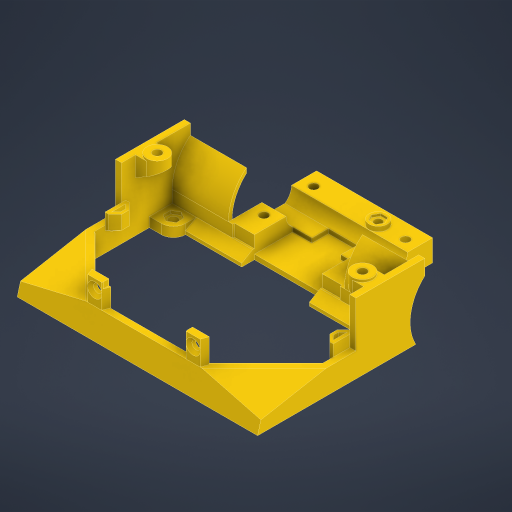
# Autodesk Inventor part: body
Saved by Autodesk Inventor 2024 (Build 280153000, 153)
## iProperties
Created: 2024-01-31
Part Number: body
Material: Všeobecné
Document SubType Name: Modeling
Designer: Simak
Density: 1 g/cm^3
Appearance: Výchozí
Author: Simak
Autodesk Inventor part; units mm, degrees
ref_plane "YZ Plane" through (0, 0, 0) normal (1, 0, 0) x (0, 1, 0)
ref_plane "XZ Plane" through (0, 0, 0) normal (0, 1, 0) x (-1, 0, 0)
ref_plane "XY Plane" through (0, 0, 0) normal (0, 0, 1) x (1, 0, 0)
sketch "Náčrt2" plane through (0, 0, 0) normal (0, 1, 0) x (-1, 0, 0)
  line L0 (0, 49.75) -> (-49.75, 49.75)
  line L1 (-49.75, 49.75) -> (-49.75, -49.75)
  line L2 (-49.75, -49.75) -> (0, -49.75)
  line L3 (-49.75, 49.75) -> (0, 0) construction
  line L4 (0, 0) -> (-49.75, -49.75) construction
  line L5 (-47.25, 49.75) -> (-47.25, -17.75)
  line L6 (-47.25, -17.75) -> (-49.75, -17.75)
  line L7 (0, 49.75) -> (0, -49.75)
  dimension "d0" = 99.5
  dimension "d1" = 67.5
  dimension "d2" = 2.5
  constraints: 16 end point, 5 perpendicular, 2 point on line, 2 vertical, 2 vertical alignment, 1 horizontal
  measures "d0" distance of L0.end L1.end
  measures "d1" distance of L5.start L5.end
  measures "d2" distance of L5.end L6.end
extrude "Vysunutí1" add sketch "Náčrt2" along normal blind 10 contours L5 L6 L1 L0
sketch "Náčrt3" plane through (49.75, 0, 49.75) normal (1, 0, 0) x (0, 0, -1)
  line L0 (67.5, 0) -> (0, 0) projected
  line L1 (67.5, 10) -> (0, 10) projected
  line L2 (0, 0) -> (0, 10) projected
  line L3 (0, 0) -> (0, -5)
  line L4 (0, -5) -> (67.5, -5) construction
  line L5 (67.5, -5) -> (67.5, 0) construction
  line L6 (0, -5) -> (4.0192, 10)
  point P0 (49.75, 0)
  point P1 (1.3397, 0)
  dimension "d8" = 5
  dimension "d9" = 75
  constraints: 8 end point, 2 perpendicular, 1 point on line, 1 vertical
  measures "d8" distance of L4.end L0.start
  measures "d9" angle of L4 L6
extrude "Vysunutí2" cut sketch "Náčrt3" against normal blind 10 contours L0 L2 L1 L6
sketch "Náčrt4" plane through (49.75, 0, -17.75) normal (1, 0, 0) x (0, 0, -1)
  line L0 (0, 10) -> (-63.4808, 10) projected
  line L1 (-60.8926, 10) -> (-63.5721, 0)
  line L2 (0, 0) -> (-66.1603, 0) projected
  line L3 (-63.4808, 10) -> (-66.1603, 0) projected
  point P0 (-17.75, 0)
  dimension "d10" = 2.5
  constraints: 2 end point, 2 point on line, 1 parallel
  measures "d10" distance between parallel lines of L3 L1
extrude "Vysunutí3" add sketch "Náčrt4" against normal up to surface (49.75 mm away)
sketch "Náčrt5" plane through (49.75, 0, -17.75) normal (1, 0, 0) x (0, 0, -1)
  line L0 (-63.4808, 10) -> (0, 10) projected
  line L1 (-25.4808, 10) -> (0, 10)
  line L2 (0, 10) -> (0, 29)
  line L3 (0, 29) -> (-25.4808, 29)
  line L4 (-25.4808, 29) -> (-25.4808, 10)
  point P0 (-17.75, 0)
  dimension "d13" = 38
  dimension "d14" = 19
  constraints: 8 end point, 2 parallel, 1 horizontal, 1 perpendicular, 1 point on line
  measures "d13" distance from line of L4 L0.start
  measures "d14" distance of L3.end L1.start
extrude "Vysunutí4" add sketch "Náčrt5" against normal up to surface (2.5 mm away)
sketch "Náčrt6" plane through (47.25, 0, -17.75) normal (-1, 0, 0) x (0, 0, 1)
  line L0 (63.5721, 0) -> (60.8926, 10) projected
  line L1 (55.5721, 1) -> (63.5721, 1)
  line L2 (63.5721, 1) -> (63.5721, 0)
  line L3 (63.5721, 0) -> (55.5721, 0)
  line L4 (55.5721, 0) -> (55.5721, 1)
  point P0 (17.75, 0)
  dimension "d17" = 1
  dimension "d18" = 8
  constraints: 8 end point, 2 parallel, 1 horizontal, 1 perpendicular
  measures "d17" distance of L3.end L1.start
  measures "d18" distance of L1.start L1.end
extrude "Vysunutí5" add sketch "Náčrt6" along normal up to surface (47.25 mm away)
sketch "Náčrt7" plane through (47.25, 0, -17.75) normal (-1, 0, 0) x (0, 0, 1)
  line L0 (60.8926, 10) -> (63.3041, 1) projected
  line L1 (62.7682, 3) -> (63.3041, 3)
  line L2 (63.3041, 3) -> (63.3041, 1)
  line L3 (63.3041, 1) -> (62.7682, 1)
  line L4 (62.7682, 1) -> (62.7682, 3)
  point P0 (17.75, 0)
  dimension "d21" = 2
  constraints: 8 end point, 2 parallel, 1 horizontal, 1 perpendicular, 1 point on line
  measures "d21" distance of L3.end L1.start
extrude "Vysunutí6" cut sketch "Náčrt7" along normal up to surface (47.25 mm away) contours L1 L2 L0
sketch "Náčrt8" plane through (0, 10, 0) normal (0, 1, 0) x (1, 0, 0)
  line L0 (49.75, -45.7308) -> (49.75, -7.7308) projected
  point P0 (0, 0)
  point P1 (24.0355, -45.7308)
  point P2 (49.75, -20.0163)
  dimension "d24" = 25.7145
  dimension "d25" = 25.7145
  constraints: 1 horizontal alignment, 1 point on line, 1 vertical alignment
  measures "d24" distance from line of L0 point (24.036, -45.731)
  measures "d25" distance of L0.start point (49.75, -20.016)
sketch "Náčrt9" plane through (49.75, 0, 48.4103) normal (1, 0, 0) x (0, 0, -1)
  line L0 (1.3397, 5) -> (0, 0) construction
  line L1 (2.6795, 10) -> (5.2677, 10) projected
  line L2 (1.3397, 5) -> (2.6795, 10) construction
  point P0 (48.4103, 0)
  constraints: 4 end point, 2 collinear
ref_plane "Pracovní rovina1" through (24.0355, 10, 45.7308) normal (-0.1788076, -0.9674997, -0.1788076) x (0.7071068, 0, -0.7071068)
sketch "Náčrt10" plane through (24.0355, 10, 45.7308) normal (-0.1788076, -0.9674997, -0.1788076) x (0.7071068, 0, -0.7071068)
  line L0 (18.1829, 17.5919) -> (-16.9957, -16.4433) projected
  line L1 (0, 0) -> (17.2355, 19.7728)
  line L2 (18.1829, 17.5919) -> (16.2882, 21.9538) projected
  line L3 (17.2355, 19.7728) -> (36.3657, 0)
  line L4 (0, 0) -> (36.3657, 0)
  point P0 (15.3408, -45.2002)
  point P1 (17.2355, 19.7728)
  point P2 (36.3657, 0)
  constraints: 6 end point, 1 coincident, 1 horizontal, 1 midpoint
extrude "Vysunutí7" cut sketch "Náčrt10" against normal blind 10
sketch "Náčrt11" plane through (24.0355, 10, 45.7308) normal (0.1788076, 0.9674997, 0.1788076) x (0.6841256, -0.2528721, 0.6841256)
  line L0 (0, 3.6603) -> (15.8603, 17.4853) projected
  line L1 (0, 0) -> (0, 3.6603) projected
  line L2 (19.7728, 17.2355) -> (0, 0) projected
  line L3 (0, 36.3657) -> (19.7728, 17.2355) projected
  line L4 (0, 32.8302) -> (0, 36.3657) projected
  line L5 (15.8603, 17.4853) -> (0, 32.8302) projected
  line L6 (0, 3.6603) -> (0, 32.8302)
  point P0 (-45.2002, 15.3408)
  constraints: 2 end point, 1 vertical
extrude "Vysunutí8" add sketch "Náčrt11" against normal blind 1.5
sketch "Náčrt13" plane through (23.7673, 8.5488, 45.4626) normal (-0.1788076, -0.9674997, -0.1788076) x (0.7071068, 0, -0.7071068)
  line L0 (17.1763, 16.5718) -> (33.2095, 0) projected
  line L1 (2.731, 0) -> (17.1763, 16.5718) projected
  line L2 (2.731, 0) -> (33.2095, 0) projected
  line L3 (33.2095, 0) -> (35.5528, -2.422)
  line L4 (43.2852, -10.1152) -> (32.8302, 0) projected
  line L5 (35.5528, -2.422) -> (0.6198, -2.422)
  line L6 (0.6198, -2.422) -> (2.731, 0)
  point P0 (15.3408, -45.2002)
  point P1 (39.216, -6.1783)
  point P2 (2.731, 0)
  point P3 (35.3336, -2.422)
  dimension "d30" = 2.422
  constraints: 6 end point, 2 collinear, 2 point on line, 1 horizontal
  measures "d30" distance between parallel lines of L2 L5
extrude "Vysunutí9" add sketch "Náčrt13" against normal up to surface contours L3 L5 L4 L2 | L2 L4 L5 L6 surface through (48.5, 10, 16) normal (0, 1, 0)
sketch "Náčrt14" plane through (0, 0, 0) normal (0, -1, 0) x (1, 0, 0)
  line L0 (47.25, 37.8221) -> (0, 37.8221) projected
  line L1 (44.25, 37.8221) -> (36.75, 37.8221)
  line L2 (36.75, 37.8221) -> (36.75, 41.8041)
  line L3 (44.25, 41.8041) -> (44.25, 37.8221)
  line L4 (49.75, 48.4103) -> (49.75, -17.75) projected
  line L5 (49.75, 48.4103) -> (0, 48.4103) projected
  arc A0 (44.25, 41.8041) -> (36.75, 41.8041) centre (40.5, 41.8041) ccw
  line L6 (47.25, 45.5541) -> (0, 45.5541) projected
  line L7 (47.25, 45.5541) -> (0, 45.5541) projected
  point P0 (0, 0)
  point P1 (36.75, 37.8221)
  point P2 (40.5, 45.5541)
  dimension "d33" = 5.5
  dimension "d35" = 7.5
  constraints: 6 end point, 3 point on circle, 2 point on line, 2 tangent, 1 centre point, 1 horizontal, 1 parallel, 1 perpendicular
  measures "d33" distance between parallel lines of L4 L3
  measures "d35" distance of L2.end L3.start
extrude "Vysunutí10" cut sketch "Náčrt14" against normal up to surface (1 mm away)
sketch "Náčrt15" plane through (47.25, 0, -17.75) normal (-1, 0, 0) x (0, 0, 1)
  circle A0 centre (-15.5, 9) radius 18.5
  line L0 (0, 0) -> (0, 29) projected
  line L1 (0, 0) -> (55.5721, 0) projected
  circle A1 centre (-15.5, 9) radius 20
  line L2 (-3, 24.6125) -> (-3, 22.6382)
  point P0 (17.75, 0)
  point P1 (0, 21.6392)
  point P2 (0, 19.0995)
  point P3 (0.6632, 0)
  point P4 (2.3606, 0)
  point P5 (0, 0.876)
  dimension "d39" = 37
  dimension "d41" = 1.5
  dimension "d38" = 15.5
  dimension "d44" = 9
  dimension "d47" = 6
  constraints: 2 end point, 1 vertical, 6 other
  measures "d38" distance from line of L0 point (-15.5, 9)
  measures "d44" distance from line of L1 point (-15.5, 9)
extrude "Vysunutí11" cut sketch "Náčrt15" against normal up to surface (2.5 mm away) contours A0 L1 L0 | L0 L1 A0
extrude "Vysunutí12" add sketch "Náčrt15" along normal blind 25 contours A0 L0 A1 L1 | A0 L2 A1 L0
sketch "Náčrt16" plane through (49.75, 29, 7.7308) normal (0, 1, 0) x (1, 0, 0)
  line L0 (-2.5, 28.4808) -> (-2.5, 25.4808) projected
  line L1 (0, 25.4808) -> (-2.5, 25.4808) projected
  line L2 (-2.5, 25.4808) -> (0, 25.4808)
  line L3 (0, 25.4808) -> (0, 28.4808)
  line L4 (0, 28.4808) -> (-2.5, 28.4808)
  line L5 (-2.5, 28.4808) -> (-2.5, 25.4808)
  point P0 (-49.75, 7.7308)
  point P1 (-2.5, 23.1202)
  constraints: 8 end point, 4 parallel, 1 horizontal, 1 perpendicular
extrude "Vysunutí13" add sketch "Náčrt16" against normal up to surface round surface about axis through (47.25, 9, -33.25) along (1, 0, 0) radius 18.5 far side no
sketch "Náčrt18" plane through (47.25, 29, 7.7308) normal (0, 1, 0) x (1, 0, 0)
  circle A0 centre (-4.75, 10) radius 4.25
  line L0 (0, 28.4808) -> (0, 0) projected
  line L1 (2.5, 0) -> (0, 0) projected
  line L2 (2.5, 28.4808) -> (2.5, 0) projected
  line L3 (2.5, 28.4808) -> (0, 28.4808) projected
  line L4 (-4.75, 5.75) -> (0, 5.75)
  line L5 (-4.75, 14.25) -> (0, 14.25)
  circle A1 centre (-4.75, 10) radius 1.75
  point P0 (-47.25, 7.7308)
  dimension "d51" = 3.5
  dimension "d52" = 2.5
  dimension "d53" = 4.75
  dimension "d54" = 10
  constraints: 4 end point, 2 centre point, 2 point on circle, 2 point on line, 1 coincident, 1 horizontal, 1 parallel, 1 perpendicular, 1 tangent
  measures "d51" diameter of A1
  measures "d52" radial gap between concentric circles of A0 A1
  measures "d53" distance from line of L0 A0.centre
  measures "d54" distance from line of L1 A0.centre
extrude "Vysunutí14" add sketch "Náčrt18" against normal blind 3.5 contours A0 | A0 L5 L0 L4
extrude "Vysunutí15" add sketch "Náčrt18" along normal blind 1 contours A0
sketch "Náčrt20" plane through (0, 0, 0) normal (0, -1, 0) x (1, 0, 0)
  line L0 (0, -14) -> (24, -14)
  line L1 (24, -14) -> (24, -49.75)
  line L2 (24, -49.75) -> (0, -49.75)
  line L3 (0, -49.75) -> (0, -14)
  line L4 (22.25, -20.75) -> (49.75, -20.75) projected
  point P0 (0, 0)
  dimension "d63" = 29
  dimension "d82" = 14
  constraints: 8 end point, 2 parallel, 1 horizontal, 1 perpendicular, 1 vertical alignment
  measures "d63" distance between parallel lines of L4 L2
  measures "d82" distance from line of point (0, 0) L0
extrude "Vysunutí16" add sketch "Náčrt20" against normal blind 9
sketch "Náčrt21" plane through (24, 0, -17.0868) normal (1, 0, 0) x (0, 0, -1)
  line L0 (12.7467, 3.9) -> (19.5797, 3.9)
  line L1 (-2.3368, 9) -> (32.6632, 9) projected
  arc A0 (19.5797, 3.9) -> (22.3018, 9) centre (16.1632, 9) ccw
  arc A1 (10.0246, 9) -> (12.7467, 3.9) centre (16.1632, 9) ccw
  line L2 (32.6632, 0) -> (32.6632, 9) projected
  point P0 (-17.0868, 0)
  point P1 (-1.6973, 9)
  dimension "d66" = 5.1
  dimension "d67" = 16.5
  dimension "d68" = 6.833
  constraints: 4 point on circle, 2 centre point, 2 end point, 2 line through centre, 2 point on line, 1 coincident, 1 concentric, 1 horizontal
  measures "d66" distance between parallel lines of L0 L1
  measures "d67" distance from line of L2 A0.centre
  measures "d68" distance of L0.start L0.end
extrude "Vysunutí17" cut sketch "Náčrt21" against normal up to next
sketch "Náčrt23" plane through (24, 0, -49.75) normal (0, 0, -1) x (-1, 0, 0)
  line L0 (0, 3.9) -> (24, 3.9) projected
  line L1 (0, 3.9) -> (24, 3.9) projected
  line L2 (18, 3.9) -> (18, 9)
  line L3 (24, 0) -> (0, 0) projected
  line L4 (24, 0) -> (24, 9) projected
  line L5 (0, 9) -> (24, 9) projected
  line L6 (0, 0) -> (0, 9) projected
  point P0 (24, 0)
  dimension "d73" = 18
  constraints: 2 end point, 2 point on line, 1 perpendicular
  measures "d73" distance between parallel lines of L6 L2
extrude "Vysunutí19" cut sketch "Náčrt23" against normal up to surface (35.75 mm away) contours L2 L5 L4 L0
sketch "Náčrt49" plane through (6, 3.9, -49.75) normal (-1, 0, 0) x (0, 0, 1)
  arc A0 (10.3614, 5.1) -> (13.0835, 0) centre (16.5, 5.1) ccw projected
  line L0 (0, 5.1) -> (10.3614, 5.1) projected
  line L1 (0, 0) -> (0, 5.1) projected
  line L2 (0, 0) -> (13.0835, 0) projected
  point P0 (49.75, -3.9)
extrude "Vysunutí48" add sketch "Náčrt49" along normal up to surface (6 mm away)
sketch "Náčrt24" plane through (0, 9, 0) normal (0, 1, 0) x (1, 0, 0)
  line L0 (22.25, 14) -> (22.25, 20.75) projected
  line L1 (47.25, 15.3894) -> (24, 15.3894) projected
  line L2 (47.25, 20.75) -> (47.25, 15.3894) projected
  line L3 (47.25, 20.75) -> (22.25, 20.75) projected
  line L4 (6, 27.1114) -> (6, 14) projected
  line L5 (24, 14.75) -> (22.25, 14.75) projected
  line L6 (24, 27.1114) -> (6, 27.1114) projected
  line L7 (24, 29.8335) -> (6, 29.8335) projected
  line L8 (24, 36.6665) -> (24, 29.8335) projected
  line L9 (24, 36.6665) -> (0, 36.6665) projected
  line L10 (0, 14) -> (0, 36.6665) projected
  line L11 (6, 29.8335) -> (6, 14) projected
  line L12 (47.25, 13.25) -> (22.25, 13.25) projected
  line L13 (22.25, 20.75) -> (22.25, 13.25) projected
  line L14 (24, 14.75) -> (24, 13.25)
  line L15 (6, 29.8335) -> (0, 29.8335)
  line L16 (6, 36.6665) -> (6, 29.8335)
  line L17 (6, 36.6665) -> (0, 36.6665)
  line L18 (22.25, 14) -> (24, 14) projected
  line L19 (24, 14) -> (24, 15.3894) projected
  line L20 (6, 14) -> (0, 14) projected
  line L21 (22.25, 14.75) -> (22.25, 14) projected
  line L22 (24, 14.75) -> (24, 27.1114) projected
  line L23 (0, 39.3886) -> (24, 39.3886) projected
  line L24 (24, 39.3886) -> (24, 49.75) projected
  line L25 (24, 49.75) -> (0, 49.75) projected
  line L26 (6, 14) -> (22.25, 14) projected
  line L27 (14, 29.8335) -> (14, 14)
  line L28 (0, 49.75) -> (0, 39.3886) projected
  point P0 (0, 0)
  point P1 (22.25, 15.3894)
  point P2 (22.25, 15.3894)
  point P3 (22.25, 13.25)
  point P4 (24, 20.75)
  dimension "d84" = 10
  constraints: 10 end point, 5 perpendicular, 5 point on line
  measures "d84" distance between parallel lines of L22 L27
extrude "Vysunutí20" cut sketch "Náčrt24" along normal up to next contours L18 L14 L12 L13 | L0 L5 L14 L18 | L0 L3 L22 L19 L5
extrude "Vysunutí21" cut sketch "Náčrt24" against normal blind 7 contours L26 L4 L6 L27 | L20 L10 L15 L11 L4 | L6 L11 L7 L27 | L15 L10 L9 L16
sketch "Náčrt31" plane through (0, 0, 0) normal (0, -1, 0) x (1, 0, 0)
  circle A0 centre (20, 39.763) radius 1.75
  arc A1 (44.25, 41.8041) -> (36.75, 41.8041) centre (40.5, 41.8041) ccw projected
  line L0 (0, 49.75) -> (49.75, 49.75) projected
  point P0 (0, 0)
  dimension "d107" = 3.5
  dimension "d108" = 20.5
  dimension "d109" = 9.987
  constraints: 1 centre point
  measures "d107" diameter of A0
  measures "d108" horizontal distance of A1.centre A0.centre
  measures "d109" distance from line of A0.centre L0
extrude "Vysunutí29" cut sketch "Náčrt31" against normal up to surface (1 mm away)
sketch "Náčrt32" plane through (0, 0, 0) normal (0, -1, 0) x (1, 0, 0)
  line L0 (0, 35.3221) -> (25, 35.3221)
  line L1 (25, 35.3221) -> (25, 37.8221)
  line L2 (36.75, 37.8221) -> (0, 37.8221) projected
  line L3 (25, 37.8221) -> (22.5, 35.3221)
  line L4 (0, 35.3221) -> (0, 37.8221)
  point P0 (0, 0)
  dimension "d112" = 25
  dimension "d113" = 2.5
  dimension "d114" = 45
  constraints: 8 end point, 2 point on line, 1 horizontal, 1 perpendicular, 1 vertical, 1 vertical alignment
  measures "d112" distance of L0.start L0.end
  measures "d113" distance of L0.end L1.end
  measures "d114" angle of L0 L3
extrude "Vysunutí30" add sketch "Náčrt32" against normal up to surface (1 mm away) contours L4 L2 L3 L0
sketch "Náčrt33" plane through (0, 9, 0) normal (0, 1, 0) x (1, 0, 0)
  circle A0 centre (19, 43.5625) radius 1.75
  circle A1 centre (19, 22.9375) radius 1.75
  line L0 (24, 27.1114) -> (14, 27.1114) projected
  line L1 (19, 27.1114) -> (19, 22.9375) construction
  line L2 (19, 43.5625) -> (19, 39.3886) construction
  line L3 (0, 39.3886) -> (24, 39.3886) projected
  line L4 (24, 39.3886) -> (24, 49.75) projected
  point P0 (0, 0)
  point P1 (6, 39.3886)
  dimension "d117" = 20.625
  dimension "d118" = 5
  dimension "d119" = 3.5
  constraints: 4 end point, 2 centre point, 2 vertical, 1 collinear, 1 equal radius, 1 midpoint, 1 point on line, 1 vertical alignment
  measures "d117" distance of L1.end L2.start
  measures "d118" distance from line of L2.start L4
  measures "d119" diameter of A1
extrude "Vysunutí31" cut sketch "Náčrt33" against normal through all
sketch "Náčrt34" plane through (0, 0, 0) normal (0, -1, 0) x (1, 0, 0)
  circle A0 centre (19, -22.9375) radius 1.75 projected
  circle A1 centre (19, -43.5625) radius 1.75 projected
  circle A2 centre (20, 39.763) radius 1.75 projected
  line L0 (0, -14) -> (0, -49.75) projected
  line L1 (0, -49.75) -> (24, -49.75) projected
  line L2 (24, -49.75) -> (24, -17.0868) projected
  line L3 (24, -17.0868) -> (49.75, -17.0868) projected
  line L4 (49.75, 48.4103) -> (49.75, -17.0868) projected
  line L5 (49.75, 48.4103) -> (0, 48.4103) projected
  line L6 (0, 35.3221) -> (0, 48.4103) projected
  line L7 (0, 35.3221) -> (22.5, 35.3221) projected
  line L8 (22.5, 35.3221) -> (25, 37.8221) projected
  line L9 (36.75, 37.8221) -> (25, 37.8221) projected
  line L10 (36.75, 37.8221) -> (36.75, 41.8041) projected
  arc A3 (44.25, 41.8041) -> (36.75, 41.8041) centre (40.5, 41.8041) ccw projected
  line L11 (44.25, 41.8041) -> (44.25, 37.8221) projected
  line L12 (47.25, 37.8221) -> (44.25, 37.8221) projected
  line L13 (47.25, -15.3894) -> (47.25, 37.8221) projected
  line L14 (47.25, -15.3894) -> (24, -15.3894) projected
  line L15 (24, -15.3894) -> (24, -14) projected
  line L16 (24, -14) -> (0, -14) projected
  circle A4 centre (42.25, -8.75) radius 1.75
  circle A5 centre (42.25, -8.75) radius 5
  line L17 (42.25, -3.75) -> (47.25, -3.75)
  line L18 (42.25, -13.75) -> (47.25, -13.75)
  line L19 (47.25, -13.25) -> (22.25, -13.25) projected
  line L20 (24, -14.75) -> (49.75, -14.75) projected
  line L21 (40.0706, -13.25) -> (40.0706, -15.3894)
  line L22 (24, -14) -> (24, -13.25)
  line L23 (42.25, -13.75) -> (40.0706, -13.75)
  line L24 (22.25, -13.25) -> (22.25, -14) projected
  line L25 (37.25, -8.75) -> (37.25, -13.25)
  point P0 (0, 0)
  dimension "d122" = 3.5
  dimension "d123" = 5
  dimension "d124" = 41
  constraints: 12 end point, 8 point on line, 5 perpendicular, 4 point on circle, 4 tangent, 2 centre point
  measures "d122" diameter of A4
  measures "d123" distance from line of L13 A4.centre
  measures "d124" distance from line of L1 A4.centre
extrude "Vysunutí32" add sketch "Náčrt34" against normal blind 4 contours L25 A5 L19 | L21 A5 L23 | L19 A5 | A5 L19 | L18 A5 L19 L13 | A5 L13 L19 | L17 L13 A5
extrude "Vysunutí33" add sketch "Náčrt34" against normal up to next contours L24 L19 L22 L16 | L22 L19 L21 L20 L15 | L20 L21 L14 L15 | L21 L23 L18 L13 L20 | L20 L13 L14 L21 | L21 A5 L23 | L19 A5 | L18 A5 L19 L13 picked at (42.7436, -13.3419)
sketch "Náčrt35" plane through (0, 4, 0) normal (0, 1, 0) x (1, 0, 0)
  circle A0 centre (42.25, 8.75) radius 1.75 projected
  line L0 (45, 7.1623) -> (42.25, 5.5746)
  line L1 (42.25, 5.5746) -> (39.5, 7.1623)
  line L2 (39.5, 7.1623) -> (39.5, 10.3377)
  line L3 (39.5, 10.3377) -> (42.25, 11.9254)
  line L4 (42.25, 11.9254) -> (45, 10.3377)
  line L5 (45, 10.3377) -> (45, 7.1623)
  point P0 (0, 0)
  dimension "d129" = 5.5
  constraints: 12 end point, 1 coincident, 1 vertical, 13 other
  measures "d129" distance between parallel lines of L2 L5
extrude "Vysunutí34" cut sketch "Náčrt35" against normal blind 1.2
sketch "Náčrt36" plane through (47.25, 25.5, 7.7308) normal (0, -1, 0) x (1, 0, 0)
  circle A0 centre (-4.75, -10) radius 1.75 projected
  line L0 (-7.5, -8.4123) -> (-4.75, -6.8246)
  line L1 (-4.75, -6.8246) -> (-2, -8.4123)
  line L2 (-2, -8.4123) -> (-2, -11.5877)
  line L3 (-2, -11.5877) -> (-4.75, -13.1754)
  line L4 (-4.75, -13.1754) -> (-7.5, -11.5877)
  line L5 (-7.5, -11.5877) -> (-7.5, -8.4123)
  point P0 (-47.25, -7.7308)
  dimension "d132" = 5.5
  constraints: 12 end point, 1 coincident, 1 vertical, 13 other
  measures "d132" distance between parallel lines of L2 L5
sketch "Náčrt37" plane through (42.5, 29, 1.9808) normal (0, 0, 1) x (1, 0, 0)
  line L0 (-4.25, 1) -> (-4.25, -3.5) projected
  line L1 (-4.25, -3) -> (4.75, -8.1962)
  line L2 (4.25, 1) -> (-4.25, 1) projected
  line L3 (7.25, 0) -> (4.75, 0) projected
  line L4 (4.75, 0) -> (4.75, -19) projected
  line L5 (7.25, -19) -> (4.75, -19) projected
  line L6 (7.25, 0) -> (7.25, -19) projected
  line L7 (7.25, 0) -> (4.75, 0) projected
  line L8 (4.75, -20) -> (4.75, -4.3875) projected
  line L9 (4.25, 1) -> (-4.25, 1) projected
  line L10 (0, 0) -> (0, -3.5) projected
  line L11 (0, -3.5) -> (0, -3.5) projected
  line L12 (0, 0) -> (0, -3.5) projected
  line L13 (0, 0) -> (0, 0) projected
  line L14 (4.75, -4.3875) -> (-18.5, -4.3875) projected
  line L15 (0, 0) -> (4.75, 0) projected
  line L16 (0, 0) -> (0, -3.5) projected
  line L17 (4.75, -3.5) -> (0, -3.5) projected
  line L18 (4.75, 0) -> (4.75, -3.5) projected
  line L19 (-4.25, -3.5) -> (0, -3.5) projected
  point P0 (-42.5, -29)
  point P1 (4.75, -9.5)
  point P2 (-3.384, -3.5)
  dimension "d139" = 3
  dimension "d142" = 60
  constraints: 3 point on line, 2 end point, 1 midpoint
  measures "d139" distance from line of L1.start L3
  measures "d142" angle of L4 L1
extrude "Vysunutí36" cut sketch "Náčrt37" against normal up to next contours L1 L19 L0
extrude "Vysunutí37" add sketch "Náčrt37" against normal up to surface (8.5 mm away) contours L19 L17 L4 L14 L1 | L14 L4 L1
sketch "Náčrt53" plane through (42.5, 30, -2.2692) normal (0, 1, 0) x (1, 0, 0)
  arc A0 (-3.384, -2.5712) -> (0, -4.25) centre (0, 0) ccw projected
  line L0 (-3.384, -4.25) -> (-3.384, -2.5712) projected
  line L1 (0, -4.25) -> (-3.384, -4.25) projected
  arc A1 (0, 4.25) -> (-3.384, 2.5712) centre (0, 0) ccw projected
  line L2 (0, 4.25) -> (-3.384, 4.25) projected
  line L3 (-3.384, 2.5712) -> (-3.384, 4.25) projected
  circle A2 centre (0, 0) radius 1.75 projected
  circle A3 centre (0, 0) radius 4.25 projected
  circle A4 centre (0, 0) radius 1.75 projected
  point P0 (-42.5, -2.2692)
extrude "Vysunutí54" cut sketch "Náčrt53" against normal up to next contours A0 L1 L0 | L3 L2 A1 | A2
extrude "Vysunutí39" cut sketch "Náčrt36" along normal blind 10 and the other way blind 1 contours A0 | L0 L1 L2 L3 L4 L5
chamfer "Zkosení3" distance 0.7 angle 45 1 edges at (40.75, 26.5, -2.2692)
sketch "Náčrt39" plane through (0, 0, 0) normal (0, -1, 0) x (1, 0, 0)
  circle A0 centre (19, -43.5625) radius 1.75 projected
  point P0 (0, 0)
  constraints: 1 coincident
hole "Díra1" at (19, 0, -43.5625) direction (0, 1, 0) diameter 3.5 depth 10.25 countersink diameter 7.5 countersink angle 90
sketch "Náčrt40" plane through (0, 10, 0) normal (0, 1, 0) x (1, 0, 0)
  line L0 (24.0355, -45.7308) -> (0, -45.7308) projected
  line L1 (17.5, -45.7308) -> (16.4809, -42.9308)
  line L2 (16.4809, -42.9308) -> (24.2691, -42.9308)
  line L3 (24.2691, -42.9308) -> (23.25, -45.7308)
  point P0 (0, 0)
  dimension "d163" = 17.5
  dimension "d164" = 5.75
  dimension "d165" = 70
  dimension "d166" = 2.8
  constraints: 6 end point, 2 point on line, 1 equal length, 1 horizontal
  measures "d163" distance of L0.end L1.start
  measures "d164" distance of L3.end L1.start
  measures "d165" angle of L0 L1
  measures "d166" distance between parallel lines of L0 L2
extrude "Vysunutí40" add sketch "Náčrt40" along normal blind 10
sketch "Náčrt41" plane through (0, 20, 0) normal (0, 1, 0) x (1, 0, 0)
  line L0 (24.2691, -42.9308) -> (16.4809, -42.9308) projected
  line L1 (17.3309, -42.9308) -> (17.3309, -45.2661)
  line L2 (16.4809, -42.9308) -> (17.5, -45.7308) projected
  line L3 (17.5, -45.7308) -> (23.25, -45.7308) projected
  line L4 (23.25, -45.7308) -> (24.2691, -42.9308) projected
  line L5 (24.2691, -42.9308) -> (16.4809, -42.9308) projected
  point P0 (0, 0)
  dimension "d169" = 0.85
  constraints: 2 end point, 2 point on line, 1 vertical
  measures "d169" distance from line of L0.end L1
extrude "Vysunutí41" cut sketch "Náčrt41" against normal blind 2.5 contours L1 L2 L0
sketch "Náčrt43" plane through (17.5, 10, 45.7308) normal (0, 0, 1) x (1, 0, 0)
  line L0 (32.25, -5) -> (6.5355, 0) projected
  line L1 (6.5355, 0) -> (5.75, 0) projected
  line L2 (5.75, 0) -> (0, 0) projected
  line L3 (0, 0) -> (-17.5, 0) projected
  line L4 (-17.5, -10) -> (-17.5, 0) projected
  line L5 (32.25, -10) -> (-17.5, -10) projected
  line L6 (32.25, -5) -> (32.25, -10) projected
  line L7 (5.75, 0) -> (0, 0) projected
  line L8 (5.75, 0) -> (5.75, 10) projected
  line L9 (0, 10) -> (5.75, 10) projected
  line L10 (0, 0) -> (0, 10) projected
  line L11 (0, 4.1599) -> (2.875, 2.5) construction
  line L12 (2.875, 2.5) -> (5.75, 4.1599) construction
  line L13 (2.875, 2.5) -> (5.75, 0) construction
  line L14 (2.875, 2.5) -> (0, 0) construction
  circle A0 centre (2.875, 5.8198) radius 2.875
  line L15 (5.75, 0) -> (5.75, 10) projected
  point P0 (-17.5, -10)
  dimension "d185" = 120
  dimension "d186" = 2.5
  constraints: 8 end point, 3 tangent, 2 equal length, 2 point on line, 1 centre point
  measures "d185" angle of L12 L11
  measures "d186" distance from line of L11.end L2
hole "Díra3" at (20.375, 15.8198, 45.7308) direction (0, 0, -1) diameter 3.5 depth 10.25 countersink diameter 6 countersink angle 90
sketch "Náčrt44" plane through (0, 10, 0) normal (0, 1, 0) x (1, 0, 0)
  line L0 (24.2691, -42.9308) -> (23.25, -45.7308) projected
  line L1 (24.0355, -45.7308) -> (23.25, -45.7308) projected
  line L2 (24.0355, -45.7308) -> (49.75, -20.0163) projected
  line L3 (49.75, -20.0163) -> (49.75, -7.7308) projected
  line L4 (49.75, -7.7308) -> (47.25, -7.7308) projected
  line L5 (47.25, -7.7308) -> (47.25, -18.976) projected
  line L6 (23.2952, -42.9308) -> (47.25, -18.976) projected
  line L7 (23.2952, -42.9308) -> (24.2691, -42.9308) projected
  line L8 (45.75, -7.8078) -> (44.25, -9.3078)
  line L9 (44.25, -9.3078) -> (44.25, -11.3078)
  line L10 (44.25, -11.3078) -> (45.75, -12.8078)
  line L11 (45.75, -12.8078) -> (45.75, -7.8078)
  line L12 (45.75, -14.5755) -> (43, -11.8255)
  line L13 (43, -8.79) -> (43, -11.8255)
  line L14 (45.75, -6.04) -> (43, -8.79)
  line L15 (45.75, -6.04) -> (47.25, -6.04)
  line L16 (47.25, -1.9808) -> (47.25, -7.7308) projected
  line L17 (49.75, -7.7308) -> (47.25, -7.7308) projected
  line L18 (49.75, 20.75) -> (49.75, -7.7308) projected
  line L19 (49.75, 20.75) -> (47.25, 20.75) projected
  line L20 (45.75, -14.5755) -> (47.25, -14.5755)
  line L21 (44.1, -11.3699) -> (44.1, -9.2456)
  line L22 (44.1, -9.2456) -> (45.9, -7.4456)
  line L23 (45.9, -7.4456) -> (45.9, -13.1699)
  line L24 (45.9, -13.1699) -> (44.1, -11.3699)
  line L25 (47.25, 20.75) -> (47.25, 6.5192) projected
  line L26 (47.25, 6.5192) -> (42.5, 6.5192) projected
  arc A0 (42.5, -1.9808) -> (42.5, 6.5192) centre (42.5, 2.2692) ccw projected
  line L27 (42.5, -1.9808) -> (47.25, -1.9808) projected
  point P0 (0, 0)
  dimension "d194" = 1.5
  dimension "d195" = 1.5
  dimension "d196" = 5
  dimension "d197" = 45
  dimension "d198" = 45
  dimension "d199" = 0.077
  dimension "d203" = 1.25
  dimension "d204" = 1.25
  dimension "d205" = 1.25
  dimension "d211" = 0.15
  constraints: 27 end point, 4 parallel, 2 point on line, 2 vertical, 2 vertical alignment, 1 horizontal, 1 perpendicular, 3 other
  measures "d194" distance between parallel lines of L9 L11
  measures "d195" distance between parallel lines of L5 L11
  measures "d196" distance of L10.end L8.start
  measures "d197" angle of L11 L10
  measures "d198" angle of L11 L8
  measures "d199" distance from line of L8.start L4
  measures "d203" distance between parallel lines of L13 L9
  measures "d204" distance between parallel lines of L12 L10
  measures "d205" distance between parallel lines of L8 L14
  measures "d211" distance between parallel lines of L9 L21
extrude "Vysunutí42" add sketch "Náčrt44" along normal blind 4.75 contours L20 L12 L13 L14 L15 L16 L5
extrude "Vysunutí43" add sketch "Náčrt44" against normal blind 1 contours L20 L12 L13 L14 L15 L16 L5 | L11 L10 L9 L8 | L21 L22 L23 L24
sketch "Náčrt45" plane through (45.75, 14.75, 14.5755) normal (0, 0, 1) x (1, 0, 0)
  line L0 (0, -5.75) -> (0, 0) projected
  line L1 (1.5, 0) -> (0, 0) projected
  line L2 (1.5, -5.75) -> (1.5, 0) projected
  line L3 (0, -5.75) -> (1.5, -5.75) projected
  line L4 (0.634, -7.25) -> (1.5, -5.75) construction
  point P0 (-45.75, -14.75)
  dimension "d214" = 120
  dimension "d215" = 1.5
  constraints: 2 end point
  measures "d214" angle of L3 L4
  measures "d215" vertical distance of L4.start L2.start
ref_plane "Pracovní rovina2" through (46.384, 7.5, 14.5755) normal (-0.8660254, 0.5, 0) x (0.5, 0.8660254, 0)
sketch "Náčrt46" plane through (46.384, 7.5, 14.5755) normal (-0.8660254, 0.5, 0) x (0.5, 0.8660254, 0)
  line L0 (-0.3929, 5.7855) -> (0.9821, 8.5355) projected
  line L1 (-0.3929, 2.75) -> (-0.3929, 5.7855) projected
  line L2 (0.9821, 0) -> (-0.3929, 2.75) projected
  line L3 (0.9821, 8.5355) -> (5.9617, 8.5355) projected
  line L4 (1.7321, 0) -> (1.7321, 8.5355) projected
  line L5 (5.9617, 0) -> (0.9821, 0) projected
  point P0 (-29.6872, 14.5755)
extrude "Vysunutí44" add sketch "Náčrt46" along normal up to surface surface through (45.125, 9, 10.3078) normal (0, -1, 0)
extrude "Vysunutí45" add sketch "Náčrt46" against normal up to surface surface through (47.25, 0, -17.75) normal (-1, 0, 0)
sketch "Náčrt47" plane through (37.25, 0, -8.75) normal (-1, 0, 0) x (0, 0, 1)
  line L0 (0, 0) -> (-4.5, 0) projected
  line L1 (0, 0) -> (0, 4) projected
  line L2 (-4.5, 4) -> (0, 4) projected
  line L3 (-4.5, 0) -> (-4.5, 4) projected
  line L4 (-5.25, 0) -> (-5.25, 9) projected
  line L5 (-4.5, 0) -> (-5.25, 0) projected
  line L6 (-4.5, 0) -> (-4.5, 9) projected
  line L7 (-4.5, 9) -> (-5.25, 9) projected
  arc A0 (-21.0835, 3.9) -> (-18.3614, 9) centre (-24.5, 9) ccw projected
  line L8 (-21.0835, 3.9) -> (-21.0835, 2) projected
  line L9 (-21.0835, 2) -> (-5.25, 2) projected
  line L10 (-5.25, 9) -> (-5.25, 2) projected
  line L11 (-18.3614, 9) -> (-5.25, 9) projected
  line L12 (-5.25, 0) -> (-41, 0) projected
  line L13 (-5.25, 0) -> (-5.25, 2) projected
  line L14 (-5.25, 2) -> (-27.9165, 2) projected
  line L15 (-4.5, 4) -> (0, 1.4019)
  line L16 (-41, 0) -> (-41, 9) projected
  line L17 (-27.9165, 2) -> (-27.9165, 3.9) projected
  arc A1 (-30.6386, 9) -> (-27.9165, 3.9) centre (-24.5, 9) ccw projected
  line L18 (-41, 9) -> (-30.6386, 9) projected
  point P0 (8.75, 0)
  dimension "d220" = 30
  constraints: 2 end point, 2 point on line
  measures "d220" angle of L2 L15
extrude "Vysunutí46" add sketch "Náčrt47" along normal up to surface (23.25 mm away) contours L0 L3 L15 L1
sketch "Náčrt48" plane through (22.25, 0, -13.25) normal (0, 0, -1) x (-1, 0, 0)
  line L0 (0, 0) -> (0, 4) projected
  line L1 (0, 0) -> (8.25, 0) projected
  line L2 (8.25, 4) -> (8.25, 0) projected
  line L3 (0, 4) -> (8.25, 4) projected
  point P0 (22.25, 0)
extrude "Vysunutí47" add sketch "Náčrt48" along normal up to next
mirror "Zrcadlit1" about plane through (0, 5, 45.7764) normal (-1, 0, 0)
sketch "Náčrt50" plane through (0, 9, 0) normal (0, 1, 0) x (1, 0, 0)
  circle A0 centre (8, 43.2692) radius 1.6
  circle A1 centre (-42.5, 2.2692) radius 1.75 projected
  circle A2 centre (8, 43.2692) radius 3.75
  line L0 (9.4434, 40.7692) -> (6.5566, 40.7692)
  line L1 (6.5566, 40.7692) -> (5.1132, 43.2692)
  line L2 (5.1132, 43.2692) -> (6.5566, 45.7692)
  line L3 (6.5566, 45.7692) -> (9.4434, 45.7692)
  line L4 (9.4434, 45.7692) -> (10.8868, 43.2692)
  line L5 (10.8868, 43.2692) -> (9.4434, 40.7692)
  point P0 (0, 0)
  dimension "d227" = 3.2
  dimension "d228" = 41
  dimension "d229" = 8
  dimension "d230" = 7.5
  dimension "d241" = 5
  constraints: 12 end point, 2 centre point, 2 coincident, 1 horizontal, 13 other
  measures "d227" diameter of A0
  measures "d228" vertical distance of A1.centre A0.centre
  measures "d229" horizontal distance of point (0, 0) A0.centre
  measures "d230" diameter of A2
  measures "d241" distance between parallel lines of L3 L0
extrude "Vysunutí49" cut sketch "Náčrt50" against normal through all contours A0
extrude "Vysunutí50" add sketch "Náčrt50" along normal blind 1 contours A2 | L0 L1 L2 L3 L4 L5
extrude "Vysunutí52" add sketch "Náčrt50" along normal blind 2 contours A2
sketch "Náčrt51" plane through (0, 0, 0) normal (0, -1, 0) x (1, 0, 0)
  circle A0 centre (8, -43.2692) radius 1.6 projected
  line L0 (9.5877, -46.0192) -> (6.4123, -46.0192)
  line L1 (6.4123, -46.0192) -> (4.8246, -43.2692)
  line L2 (4.8246, -43.2692) -> (6.4123, -40.5192)
  line L3 (6.4123, -40.5192) -> (9.5877, -40.5192)
  line L4 (9.5877, -40.5192) -> (11.1754, -43.2692)
  line L5 (11.1754, -43.2692) -> (9.5877, -46.0192)
  point P0 (0, 0)
  dimension "d235" = 5.5
  constraints: 12 end point, 1 coincident, 1 horizontal, 13 other
  measures "d235" distance between parallel lines of L3 L0
extrude "Vysunutí51" cut sketch "Náčrt51" against normal blind 6 contours A0 | L0 L1 L2 L3 L4 L5
chamfer "Zkosení4" distance 0.7 angle 45 1 edges at (6.4, 6, -43.2692)
